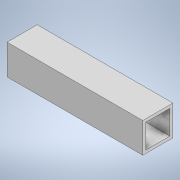
# Autodesk Inventor part: finger_straight_hollow
Saved by Autodesk Inventor 2021 (Build 250183000, 183)
## iProperties
Created: 2021-03-11
Part Number: finger_straight_hollow
Material: Generic
Document SubType Name: Modeling
Designer: Charlie
Density: 1 g/cm^3
Appearance: Default
Author: Charlie
Autodesk Inventor part; units mm, degrees
ref_plane "YZ Plane" through (0, 0, 0) normal (1, 0, 0) x (0, 1, 0)
ref_plane "XZ Plane" through (0, 0, 0) normal (0, 1, 0) x (-1, 0, 0)
ref_plane "XY Plane" through (0, 0, 0) normal (0, 0, 1) x (1, 0, 0)
sketch "Sketch1" plane through (0, 0, 0) normal (0, 1, 0) x (-1, 0, 0)
  line L0 (-15, 10) -> (15, 10)
  line L1 (15, 10) -> (15, -10)
  line L2 (15, -10) -> (-15, -10)
  line L3 (-15, -10) -> (-15, 10)
  line L4 (-15, 10) -> (15, -10) construction
  line L5 (15, 10) -> (-15, -10) construction
  line L6 (15, 10) -> (45, 10)
  line L7 (45, 10) -> (45, -10)
  line L8 (45, -10) -> (15, -10)
  line L9 (15, -10) -> (15, 10)
  line L10 (45, 10) -> (75, 10)
  line L11 (75, 10) -> (75, -10)
  line L12 (75, -10) -> (45, -10)
  line L13 (45, -10) -> (45, 10)
  point P0 (0, 0)
  point P1 (15, -10)
  dimension "d0" = 30
  dimension "d1" = 20
  dimension "d2" = 30
  dimension "d3" = 30
  dimension "d4" = 20
  dimension "d5" = 30
  constraints: 28 end point, 6 parallel, 3 horizontal, 3 perpendicular, 2 midpoint
  measures "d0" distance of L1.end L2.end
  measures "d1" distance of L0.end L1.end
  measures "d2" distance of L7.end L8.end
  measures "d3" distance of L11.end L12.end
  measures "d4" distance of L10.end L11.end
  measures "d5" distance between parallel lines of L1 L7
extrude "Extrusion1" add sketch "Sketch1" along normal blind 20
shell "Shell1" thickness 2 removed faces 2 at (15, 6.6667, 3.3333) at (-75, 6.6667, -3.3333)
body "Solid1"
